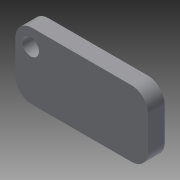
# Autodesk Inventor part: Keychain_Bowen
Saved by Autodesk Inventor 2014 (Build 180170000, 170)
## iProperties
Created: 2014-09-09
Part Number: Keychain_Bowen
Material: Generic
Document SubType Name: Modeling
Designer: 1750019
Density: 1 g/cm^3
Appearance: Default
Author: 1750019
Autodesk Inventor part; units mm, degrees
ref_plane "YZ Plane" through (0, 0, 0) normal (1, 0, 0) x (0, 1, 0)
ref_plane "XZ Plane" through (0, 0, 0) normal (0, 1, 0) x (-1, 0, 0)
ref_plane "XY Plane" through (0, 0, 0) normal (0, 0, 1) x (1, 0, 0)
sketch "Sketch1" plane through (0, 0, 0) normal (0, 0, 1) x (1, 0, 0)
  line L0 (0, 0) -> (25.4, 0)
  line L1 (25.4, 0) -> (25.4, -12.7)
  line L2 (25.4, -12.7) -> (0, -12.7)
  line L3 (0, -12.7) -> (0, 0)
  dimension "d0" = 25.4
  dimension "d1" = 12.7
  constraints: 8 end point, 2 perpendicular, 1 horizontal, 1 parallel
  measures "d0" distance of L0.start L0.end
  measures "d1" distance of L0.end L1.end
extrude "Extrusion1" add sketch "Sketch1" along normal blind 3.175
hole "Hole1" at (2.933, -3.2804, 3.175) direction (0, 0, -1) diameter 3.175 depth 3.175 tip angle 118
fillet "Fillet1" radius 3.175 4 edges at (25.4, 0, 1.5875) (0, 0, 1.5875) (0, -12.7, 1.5875) (25.4, -12.7, 1.5875)
body "Solid1"
